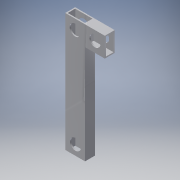
# Autodesk Inventor part: arm
Saved by Autodesk Inventor 2016 (Build 200138000, 138)
## iProperties
Created: 2016-01-27
Part Number: arm
Material: Aluminum 6061
Document SubType Name: Modeling
Designer: 278648
Density: 2.7 g/cm^3
Appearance: Aluminum - Flat
Mass: 392.719 g
Surface Area: 942.707 cm^2
Volume: 145.451 cm^3
Author: 278648
Autodesk Inventor part; units mm, degrees
ref_plane "YZ Plane" through (0, 0, 0) normal (1, 0, 0) x (0, 1, 0)
ref_plane "XZ Plane" through (0, 0, 0) normal (0, 1, 0) x (-1, 0, 0)
ref_plane "XY Plane" through (0, 0, 0) normal (0, 0, 1) x (1, 0, 0)
sketch "Sketch1" plane through (0, 0, 0) normal (0, 1, 0) x (-1, 0, 0)
  line L0 (0, 0) -> (50.8, 0)
  line L1 (50.8, 0) -> (50.8, -25.4)
  line L2 (50.8, -25.4) -> (0, -25.4)
  line L3 (0, -25.4) -> (0, 0)
  line L4 (47.625, -3.1826) -> (3.175, -3.1826)
  line L5 (3.175, -3.1826) -> (3.175, -22.225)
  line L6 (3.175, -22.225) -> (47.625, -22.225)
  line L7 (47.625, -22.225) -> (47.625, -3.1826)
  dimension "d0" = 50.8
  dimension "d1" = 25.4
  dimension "d2" = 3.175
  dimension "d3" = 3.1826
  dimension "d4" = 3.175
  dimension "d5" = 3.175
  constraints: 16 end point, 4 parallel, 2 horizontal, 2 perpendicular
  measures "d0" distance between parallel lines of L3 L1
  measures "d1" distance between parallel lines of L0 L2
  measures "d2" distance between parallel lines of L2 L6
  measures "d3" distance between parallel lines of L0 L4
  measures "d4" distance between parallel lines of L3 L5
  measures "d5" distance between parallel lines of L1 L7
extrude "Extrusion1" add sketch "Sketch1" along normal blind 304.8
sketch "Sketch2" plane through (0, 0, 0) normal (1, 0, 0) x (0, 0, -1)
  line L0 (25.4, 0) -> (25.4, 304.8) projected
  line L1 (0, 304.8) -> (25.4, 304.8)
  line L2 (25.4, 304.8) -> (25.4, 254)
  line L3 (25.4, 254) -> (0, 254)
  line L4 (0, 254) -> (0, 304.8)
  line L5 (3.1826, 0) -> (3.1826, 304.8) projected
  line L6 (3.1826, 301.7936) -> (22.225, 301.7936)
  line L7 (22.225, 301.7936) -> (22.225, 257.175)
  line L8 (22.225, 257.175) -> (3.1826, 257.175)
  line L9 (3.1826, 257.175) -> (3.1826, 301.7936)
  point P0 (0, 0)
  dimension "d8" = 50.8
  dimension "d9" = 3.175
  dimension "d10" = 3.175
  constraints: 16 end point, 4 parallel, 2 horizontal, 2 perpendicular, 2 point on line
  measures "d8" distance between parallel lines of L1 L3
  measures "d9" distance between parallel lines of L8 L3
  measures "d10" distance between parallel lines of L0 L7
extrude "Extrusion2" add sketch "Sketch2" along normal blind 50.8 contours L3 L5 L8 L7 L6 L1 L0 | L3 L4 L1 L5
sketch "Sketch3" plane through (0, 0, -25.4) normal (0, 0, -1) x (-1, 0, 0)
  circle A0 centre (-25.4, 280.6907) radius 14.2875
  line L0 (-50.8, 254) -> (-50.8, 304.8) projected
  point P0 (0, 0)
  dimension "d13" = 25.4
  dimension "d14" = 28.575
  constraints: 1 centre point
  measures "d13" distance from line of L0 A0.centre
  measures "d14" diameter of A0
extrude "Extrusion3" cut sketch "Sketch3" against normal through all
sketch "Sketch4" plane through (0, 0, -25.4) normal (0, 0, -1) x (-1, 0, 0)
  circle A0 centre (24.6023, 25.4) radius 14.2875
  line L0 (50.8, 0) -> (0, 0) projected
  dimension "d17" = 25.4
  dimension "d18" = 28.575
  constraints: 1 centre point
  measures "d17" distance from line of L0 A0.centre
  measures "d18" diameter of A0
extrude "Extrusion4" cut sketch "Sketch4" against normal through all
sketch "Sketch5" plane through (0, 0, -25.4) normal (0, 0, -1) x (-1, 0, 0)
  circle A0 centre (25.4, 279.4) radius 14.2875
  line L0 (50.8, 304.8) -> (-50.8, 304.8) projected
  line L1 (50.8, 0) -> (50.8, 304.8) projected
  point P0 (0, 0)
  dimension "d21" = 25.4
  dimension "d22" = 28.575
  dimension "d23" = 25.4
  constraints: 1 centre point
  measures "d21" distance from line of L0 A0.centre
  measures "d22" diameter of A0
  measures "d23" distance from line of L1 A0.centre
extrude "Extrusion5" cut sketch "Sketch5" against normal blind 25.4
body "Solid1"
